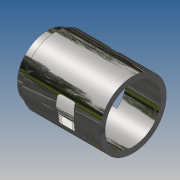
# Autodesk Inventor part: Zylinderbuchse_ra8846s
Saved by Autodesk Inventor 2021 (Build 250183000, 183)
## iProperties
Created: 2020-12-16
Part Number: Zylinderbuchse_ra8846s
Material: Stahl, Guss
Document SubType Name: Modeling
Designer: Ricardo
Density: 7.85 g/cm^3
Appearance: Halbpoliert
Mass: 7.87408 g
Surface Area: 18.401 cm^2
Volume: 1.00307 cm^3
Author: Ricardo Aviles
Revision Number: Rev00
Autodesk Inventor part; units mm, degrees
ref_plane "YZ-Ebene" through (0, 0, 0) normal (1, 0, 0) x (0, 1, 0)
ref_plane "XY-Ebene" through (0, 0, 0) normal (0, 0, 1) x (1, 0, 0)
sketch "Skizze1" plane through (0, 0, 0) normal (0, 0, 1) x (1, 0, 0)
  line L0 (-4, 0) -> (24, 0) projected
  line L1 (0, -1.56) -> (0, 9.36) projected
  line L2 (0, 7) -> (2, 7)
  line L3 (2, 7) -> (2, 7.8)
  line L4 (2, 7.8) -> (20, 7.8)
  line L5 (20, 7.8) -> (20, 6.5)
  line L6 (20, 6.5) -> (0, 6.5)
  line L7 (0, 7) -> (0, 6.5)
  point P0 (0, 0)
  dimension "d0" = 6.5
  dimension "d1" = 7.8
  dimension "d2" = 7
  dimension "d3" = 2
  dimension "d4" = 20
  constraints: 12 end point, 5 perpendicular, 2 point on line, 1 horizontal
  measures "d0" distance from line of L0 L5.end
  measures "d1" distance from line of L0 L4.end
  measures "d2" distance from line of L0 L2.start
  measures "d3" distance of L2.start L2.end
  measures "d4" horizontal distance of L4.end L2.start
revolve "Umdrehung1" add sketch "Skizze1" angle 360 about axis through (-10, 0, 0) along (1, 0, 0)
ref_plane "Arbeitsebene1" through (11, 7.8, 0) normal (0, 1, 0) x (-1, 0, 0)
sketch "Skizze2" plane through (11, 7.8, 0) normal (0, 1, 0) x (-1, 0, 0)
  line L0 (9, 7.8) -> (9, -7.8) projected
  line L1 (-9, 7.8) -> (-9, -7.8) projected
  line L2 (9, -7.8) -> (-9, -7.8) projected
  line L3 (9, 7.8) -> (-9, 7.8) projected
  line L4 (2.5, 10) -> (2.5, -10)
  line L5 (2.5, -10) -> (-1, -10)
  line L6 (-1, -10) -> (-1, 10)
  line L7 (-1, 10) -> (2.5, 10)
  line L8 (11, 7) -> (11, -7) projected
  line L9 (15, 0) -> (-13, 0) projected
  point P0 (11, 0)
  dimension "d6" = 20
  dimension "d7" = 3.5
  dimension "d8" = 8.5
  constraints: 8 end point, 3 perpendicular, 1 vertical, 1 other
  measures "d6" distance of L5.end L6.end
  measures "d7" distance of L4.end L5.end
  measures "d8" distance from line of L8 L4.end
extrude "Extrusion1" cut sketch "Skizze2" against normal blind 3.5 contours L4 L9 L6 L3 | L3 L6 L7 L4 | L4 L2 L6 L9 | L4 L5 L6 L2
sketch "Skizze3" plane through (0, 0, 0) normal (0, 0, 1) x (1, 0, 0)
  point P0 (0, 0)
sketch "Skizze4" plane through (0, 0, 0) normal (1, 0, 0) x (0, 1, 0)
  point P0 (0, 0)
sketch "Skizze5" plane through (0, 0, 0) normal (0, 0, 1) x (1, 0, 0)
  point P0 (0, 0)
sketch "Skizze6" plane through (0, 0, 0) normal (0, 0, 1) x (1, 0, 0)
  point P0 (0, 0)
sketch "Skizze7" plane through (0, 0, 0) normal (0, 0, 1) x (1, 0, 0)
  line L0 (2, -7.8) -> (20, -7.8) projected
  line L1 (12.982, -10.982) -> (6.618, -4.618)
  line L2 (15.1033, -8.8607) -> (12.982, -10.982)
  line L3 (6.618, -4.618) -> (8.7393, -2.4967)
  line L4 (15.1033, -8.8607) -> (8.7393, -2.4967)
  line L5 (20, -6.5) -> (20, 6.5) projected
  line L6 (-4, 0) -> (24, 0) projected
  point P0 (0, 0)
  point P1 (9.8, -7.8)
  dimension "d12" = 9
  dimension "d13" = 3
  dimension "d14" = 10.2
  dimension "d19" = 9
  dimension "d20" = 3
  dimension "d21" = 45
  constraints: 8 end point, 1 midpoint, 1 point on line
  measures "d12" distance of L1.start L1.end
  measures "d13" distance of L2.start L1.start
  measures "d14" distance from line of L5 point (9.8, -7.8)
  measures "d19" distance between parallel lines of L2 L3
  measures "d20" distance of L1.end L3.end
  measures "d21" angle of L0 L4
revolve "Umdrehung2" cut sketch "Skizze7" angle 45 mid plane about axis through (-10, 0, 0) along (1, 0, 0)
fillet "Rundung1" radius 0.6 4 edges at (13.3926, -6.6057, -2.7362) (13.3926, -6.6057, 2.7362) (9.15, -6.6057, 2.7362) (9.15, -6.6057, -2.7362)
